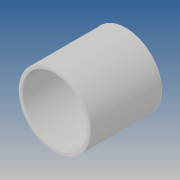
# Autodesk Inventor part: douille
Saved by Autodesk Inventor 2019 (Build 230136000, 136)
## iProperties
Created: 2018-05-05
Part Number: douille
Material: Générique
Document SubType Name: Modeling
Designer: Theo
Density: 1 g/cm^3
Appearance: Par défaut
Author: Theo
Autodesk Inventor part; units mm, degrees
ref_plane "YZ Plane" through (0, 0, 0) normal (1, 0, 0) x (0, 1, 0)
ref_plane "XZ Plane" through (0, 0, 0) normal (0, 1, 0) x (-1, 0, 0)
ref_plane "XY Plane" through (0, 0, 0) normal (0, 0, 1) x (1, 0, 0)
sketch "Esquisse1" plane through (0, 0, 0) normal (1, 0, 0) x (0, 1, 0)
  line L0 (0, 0) -> (0, -39.3305)
  line L1 (12.5, -0.25) -> (12.5, -25)
  line L2 (12.25, 0) -> (11.5, 0)
  line L3 (11.25, -0.25) -> (11.25, -25)
  arc A0 (11.5, 0) -> (11.25, -0.25) centre (11.5, -0.25) ccw
  arc A1 (12.5, -0.25) -> (12.25, 0) centre (12.25, -0.25) ccw
  line L4 (11, -0.25) -> (11, -25) construction
  line L5 (11.25, -25) -> (12.5, -25)
  dimension "d0" = 25
  dimension "d2" = 0.25
  dimension "d3" = 0.25
  dimension "d5" = 0.25
  dimension "d6" = 22
  dimension "d7" = 25
  constraints: 12 end point, 4 point on circle, 4 tangent, 4 vertical, 3 horizontal alignment, 2 centre point, 2 horizontal
  measures "d0" diameter of L1 L0
  measures "d2" radius of A0
  measures "d3" radius of A1
  measures "d5" distance between parallel lines of L3 L4
  measures "d6" diameter of L4 L0
  measures "d7" distance between parallel lines of L5 L2
revolve "Révolution1" add sketch "Esquisse1" angle 360 about axis through (0, 0, 0) along (0, 0, -1)
